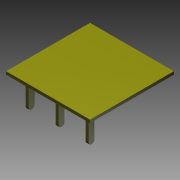
# Autodesk Inventor part: UB216SKG035D-NR
Saved by Autodesk Inventor 2015 SP1 (Build 190203100, 203)
## iProperties
Category: Electrical
Company: Autodesk Inc.
Created: 2014-12-16
Part Number: UB216SKG035D-NR
Catalog Web Link: http://www.nkkswitches.com/
Description: PC and Snap-in Mount Non-Illuminated Pushbuttons_ni_pole-Non-Illuminated Pushbuttons - Series UB2
Vendor: NKK Switches
Document SubType Name: Modeling
Designer: Autodesk Inc.
Manufacturer: NKKSWITCHES
Mass: 0.110173 g
Surface Area: 4.7726 cm^2
Volume: 0.110173 cm^3
Density: 1 g/cm^3
Material: Generic
Appearance: PSOLRGB-255-255-0
Title: UB21G03-5Dni_pole
Author: Autodesk Inc.
Comments: Non-Illuminated Pushbuttons - Series UB2
Autodesk Inventor part; units mm, degrees
sketch "Sketch_1" plane through (0, 0, 0) normal (0, 1, 0) x (-1, 0, 0)
  line L0 (7.112, -7.112) -> (7.112, 7.112)
  line L1 (7.112, 7.112) -> (-7.112, 7.112)
  line L2 (-7.112, 7.112) -> (-7.112, -7.112)
  line L3 (-7.112, -7.112) -> (7.112, -7.112)
  constraints: 8 end point
extrude "Extrusion1" add sketch "Sketch_1" along normal blind 0.508
sketch "Sketch_10" plane through (-5.08, 0, 0) normal (1, 0, 0) x (0, 0, -1)
  arc A0 (-5.5753, -4.5085) -> (-5.08, -5.0038) centre (-5.08, -4.5085) ccw
  arc A1 (-5.08, -5.0038) -> (-4.5847, -4.5085) centre (-5.08, -4.5085) ccw
  line L0 (-4.5847, -4.5085) -> (-4.5847, 0.508)
  line L1 (-4.5847, 0.508) -> (-5.5753, 0.508)
  line L2 (-5.5753, 0.508) -> (-5.5753, -4.5085)
  constraints: 6 end point, 4 point on circle, 2 centre point
extrude "Extrusion2" add sketch "Sketch_10" along normal mid plane 0.508
sketch "Sketch_12" plane through (0, 0, 0) normal (1, 0, 0) x (0, 1, 0)
  arc A0 (-4.5085, 5.5753) -> (-5.0038, 5.08) centre (-4.5085, 5.08) ccw
  arc A1 (-5.0038, 5.08) -> (-4.5085, 4.5847) centre (-4.5085, 5.08) ccw
  line L0 (-4.5085, 4.5847) -> (0.508, 4.5847)
  line L1 (0.508, 4.5847) -> (0.508, 5.5753)
  line L2 (0.508, 5.5753) -> (-4.5085, 5.5753)
  constraints: 6 end point, 4 point on circle, 2 centre point
extrude "Extrusion3" add sketch "Sketch_12" along normal mid plane 0.508
sketch "Sketch_14" plane through (5.08, 0, 0) normal (1, 0, 0) x (0, 0, -1)
  arc A0 (-5.5753, -4.5085) -> (-5.08, -5.0038) centre (-5.08, -4.5085) ccw
  arc A1 (-5.08, -5.0038) -> (-4.5847, -4.5085) centre (-5.08, -4.5085) ccw
  line L0 (-4.5847, -4.5085) -> (-4.5847, 0.508)
  line L1 (-4.5847, 0.508) -> (-5.5753, 0.508)
  line L2 (-5.5753, 0.508) -> (-5.5753, -4.5085)
  constraints: 6 end point, 4 point on circle, 2 centre point
extrude "Extrusion4" add sketch "Sketch_14" along normal mid plane 0.508
ref_plane "pole_to_body_XY" through (0, 0.508, 0) normal (0, 1, 0) x (1, 0, 0)
ref_plane "pole_to_body_YZ" through (0, 0.508, 0) normal (1, 0, 0) x (0, 0, -1)
ref_plane "pole_to_body_ZX" through (0, 0.508, 0) normal (0, 0, -1) x (0, 1, 0)
body "Solid1"
